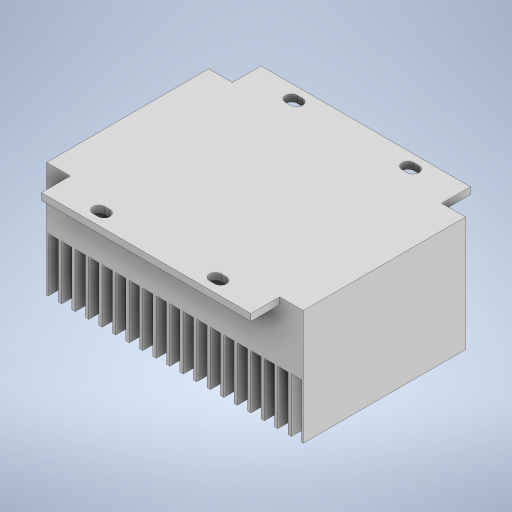
# Autodesk Inventor part: N0039 ERAM-0.01-1G-2W
Saved by Autodesk Inventor 2023 (Build 270158000, 158)
## iProperties
Created: 2023-10-03
Part Number: N0039 ERAM-0.01-1G-2W
Material: 一般
Document SubType Name: Modeling
Designer: 310611102
Density: 1 g/cm^3
Appearance: 預設
Author: 310611102
Autodesk Inventor part; units mm, degrees
ref_plane "YZ Plane" through (0, 0, 0) normal (1, 0, 0) x (0, 1, 0)
ref_plane "XZ Plane" through (0, 0, 0) normal (0, 1, 0) x (-1, 0, 0)
ref_plane "XY Plane" through (0, 0, 0) normal (0, 0, 1) x (1, 0, 0)
sketch "Sketch1" plane through (0, 0, 0) normal (0, 0, 1) x (1, 0, 0)
  line L0 (-38, 16) -> (38, 16)
  line L1 (38, 16) -> (38, -16)
  line L2 (38, -16) -> (-38, -16)
  line L3 (-38, -16) -> (-38, 16)
  line L4 (-38, 16) -> (38, -16) construction
  line L5 (38, 16) -> (-38, -16) construction
  point P0 (0, 0)
  dimension "d0" = 76
  dimension "d1" = 32
  constraints: 12 end point, 2 midpoint, 2 parallel, 1 horizontal, 1 perpendicular
  measures "d0" distance of L0.start L0.end
  measures "d1" distance of L0.end L1.end
extrude "Extrusion1" add sketch "Sketch1" along normal mid plane 48
sketch "Sketch2" plane through (-38, 16, 24) normal (0, 1, 0) x (1, 0, 0)
  line L0 (69, -8.5) -> (7, -8.5)
  line L1 (7, -8.5) -> (7, 56.5)
  line L2 (7, 56.5) -> (69, 56.5)
  line L3 (69, 56.5) -> (69, -8.5)
  line L4 (69, -8.5) -> (7, 56.5) construction
  line L5 (7, -8.5) -> (69, 56.5) construction
  line L6 (7, 48) -> (0, 48)
  line L7 (0, 48) -> (0, 0)
  line L8 (0, 0) -> (7, 0)
  line L9 (7, 0) -> (7, 48)
  line L10 (7, 48) -> (0, 0) construction
  line L11 (0, 48) -> (7, 0) construction
  line L12 (76, 48) -> (69, 48)
  line L13 (69, 48) -> (69, 0)
  line L14 (69, 0) -> (76, 0)
  line L15 (76, 0) -> (76, 48)
  line L16 (76, 48) -> (69, 0) construction
  line L17 (69, 48) -> (76, 0) construction
  line L18 (0, 48) -> (76, 48) projected
  line L19 (76, 48) -> (76, 0) projected
  line L20 (20, -4.5) -> (21.5, -4.5) construction
  line L21 (20, -6.25) -> (21.5, -6.25)
  line L22 (21.5, -2.75) -> (20, -2.75)
  arc A0 (20, -2.75) -> (20, -6.25) centre (20, -4.5) ccw
  arc A1 (21.5, -6.25) -> (21.5, -2.75) centre (21.5, -4.5) ccw
  line L23 (28.4806, 24) -> (38, 24) construction
  line L24 (38, 24) -> (38, 34.5741) construction
  line L25 (20, 52.5) -> (21.5, 52.5) construction
  line L26 (20, 54.25) -> (21.5, 54.25)
  line L27 (21.5, 50.75) -> (20, 50.75)
  arc A2 (20, 54.25) -> (20, 50.75) centre (20, 52.5) ccw
  arc A3 (21.5, 50.75) -> (21.5, 54.25) centre (21.5, 52.5) ccw
  line L28 (56, -4.5) -> (54.5, -4.5) construction
  line L29 (56, -6.25) -> (54.5, -6.25)
  line L30 (54.5, -2.75) -> (56, -2.75)
  arc A4 (56, -6.25) -> (56, -2.75) centre (56, -4.5) ccw
  arc A5 (54.5, -2.75) -> (54.5, -6.25) centre (54.5, -4.5) ccw
  line L31 (56, 54.25) -> (54.5, 54.25)
  line L32 (56, 52.5) -> (54.5, 52.5) construction
  line L33 (54.5, 50.75) -> (56, 50.75)
  arc A6 (54.5, 54.25) -> (54.5, 50.75) centre (54.5, 52.5) ccw
  arc A7 (56, 50.75) -> (56, 54.25) centre (56, 52.5) ccw
  point P0 (3.5, 24)
  point P1 (72.5, 24)
  point P2 (20.75, -4.5)
  point P3 (20.75, 52.5)
  point P4 (55.25, -4.5)
  point P5 (55.25, 52.5)
  point P6 (23.25, -4.5)
  point P7 (18.25, -4.5)
  point P8 (20.75, -6.25)
  point P9 (20.75, -2.75)
  point P10 (20.75, 52.5)
  point P11 (55.25, -4.5)
  point P12 (69, 48)
  point P13 (7, 48)
  point P14 (7, 0)
  dimension "d4" = 65
  dimension "d5" = 62
  dimension "d6" = 5
  dimension "d7" = 3.5
  dimension "d8" = 57
  dimension "d12" = 36
  constraints: 72 end point, 21 symmetric about line, 18 point on circle, 11 midpoint, 8 centre point, 7 parallel, 5 horizontal, 4 tangent, 3 collinear, 3 perpendicular, 2 point on line, 1 vertical, 6 other
  measures "d4" distance between parallel lines of L0 L2
  measures "d5" distance of L1.end L2.end
  measures "d6" distance of point (23.25, -4.5) point (18.25, -4.5)
  measures "d7" distance of point (20.75, -6.25) point (20.75, -2.75)
  measures "d8" distance of point (20.75, 52.5) point (20.75, -4.5)
  measures "d12" distance of L28.start L20.start
extrude "Extrusion2" add sketch "Sketch2" along normal blind 2
sketch "Sketch3" plane through (0, 0, 24) normal (0, 0, 1) x (1, 0, 0)
  line L0 (38, -16) -> (-38, -16) projected
  line L1 (-1.5, 0) -> (1.5, 0)
  line L2 (1.5, 0) -> (1.5, -16)
  line L3 (1.5, -16) -> (-1.5, -16)
  line L4 (-1.5, -16) -> (-1.5, 0)
  line L5 (-1.5, 0) -> (1.5, -16) construction
  line L6 (1.5, 0) -> (-1.5, -16) construction
  line L7 (-5.5, 0) -> (-2.5, 0)
  line L8 (-2.5, 0) -> (-2.5, -16)
  line L9 (-2.5, -16) -> (-5.5, -16)
  line L10 (-5.5, -16) -> (-5.5, 0)
  line L11 (-5.5, 0) -> (-2.5, -16) construction
  line L12 (-2.5, 0) -> (-5.5, -16) construction
  line L13 (-9.5, 0) -> (-6.5, 0)
  line L14 (-6.5, 0) -> (-6.5, -16)
  line L15 (-6.5, -16) -> (-9.5, -16)
  line L16 (-9.5, -16) -> (-9.5, 0)
  line L17 (-9.5, 0) -> (-6.5, -16) construction
  line L18 (-6.5, 0) -> (-9.5, -16) construction
  line L19 (-13.5, 0) -> (-10.5, 0)
  line L20 (-10.5, 0) -> (-10.5, -16)
  line L21 (-10.5, -16) -> (-13.5, -16)
  line L22 (-13.5, -16) -> (-13.5, 0)
  line L23 (-13.5, 0) -> (-10.5, -16) construction
  line L24 (-10.5, 0) -> (-13.5, -16) construction
  line L25 (-17.5, 0) -> (-14.5, 0)
  line L26 (-14.5, 0) -> (-14.5, -16)
  line L27 (-14.5, -16) -> (-17.5, -16)
  line L28 (-17.5, -16) -> (-17.5, 0)
  line L29 (-17.5, 0) -> (-14.5, -16) construction
  line L30 (-14.5, 0) -> (-17.5, -16) construction
  line L31 (2.5, 0) -> (5.5, 0)
  line L32 (5.5, 0) -> (5.5, -16)
  line L33 (5.5, -16) -> (2.5, -16)
  line L34 (2.5, -16) -> (2.5, 0)
  line L35 (2.5, 0) -> (5.5, -16) construction
  line L36 (5.5, 0) -> (2.5, -16) construction
  line L37 (-1.5, 0) -> (1.5, 0)
  line L38 (1.5, 0) -> (1.5, -16)
  line L39 (1.5, -16) -> (-1.5, -16)
  line L40 (-1.5, -16) -> (-1.5, 0)
  line L41 (-1.5, 0) -> (1.5, -16) construction
  line L42 (1.5, 0) -> (-1.5, -16) construction
  line L43 (-5.5, 0) -> (-2.5, 0)
  line L44 (-2.5, 0) -> (-2.5, -16)
  line L45 (-2.5, -16) -> (-5.5, -16)
  line L46 (-5.5, -16) -> (-5.5, 0)
  line L47 (-5.5, 0) -> (-2.5, -16) construction
  line L48 (-2.5, 0) -> (-5.5, -16) construction
  line L49 (-9.5, 0) -> (-6.5, 0)
  line L50 (-6.5, 0) -> (-6.5, -16)
  line L51 (-6.5, -16) -> (-9.5, -16)
  line L52 (-9.5, -16) -> (-9.5, 0)
  line L53 (-9.5, 0) -> (-6.5, -16) construction
  line L54 (-6.5, 0) -> (-9.5, -16) construction
  line L55 (-13.5, 0) -> (-10.5, 0)
  line L56 (-10.5, 0) -> (-10.5, -16)
  line L57 (-10.5, -16) -> (-13.5, -16)
  line L58 (-13.5, -16) -> (-13.5, 0)
  line L59 (-13.5, 0) -> (-10.5, -16) construction
  line L60 (-10.5, 0) -> (-13.5, -16) construction
  line L61 (6.5, 0) -> (9.5, 0)
  line L62 (9.5, 0) -> (9.5, -16)
  line L63 (9.5, -16) -> (6.5, -16)
  line L64 (6.5, -16) -> (6.5, 0)
  line L65 (6.5, 0) -> (9.5, -16) construction
  line L66 (9.5, 0) -> (6.5, -16) construction
  line L67 (2.5, 0) -> (5.5, 0)
  line L68 (5.5, 0) -> (5.5, -16)
  line L69 (5.5, -16) -> (2.5, -16)
  line L70 (2.5, -16) -> (2.5, 0)
  line L71 (2.5, 0) -> (5.5, -16) construction
  line L72 (5.5, 0) -> (2.5, -16) construction
  line L73 (-1.5, 0) -> (1.5, 0)
  line L74 (1.5, 0) -> (1.5, -16)
  line L75 (1.5, -16) -> (-1.5, -16)
  line L76 (-1.5, -16) -> (-1.5, 0)
  line L77 (-1.5, 0) -> (1.5, -16) construction
  line L78 (1.5, 0) -> (-1.5, -16) construction
  line L79 (-5.5, 0) -> (-2.5, 0)
  line L80 (-2.5, 0) -> (-2.5, -16)
  line L81 (-2.5, -16) -> (-5.5, -16)
  line L82 (-5.5, -16) -> (-5.5, 0)
  line L83 (-5.5, 0) -> (-2.5, -16) construction
  line L84 (-2.5, 0) -> (-5.5, -16) construction
  line L85 (-9.5, 0) -> (-6.5, 0)
  line L86 (-6.5, 0) -> (-6.5, -16)
  line L87 (-6.5, -16) -> (-9.5, -16)
  line L88 (-9.5, -16) -> (-9.5, 0)
  line L89 (-9.5, 0) -> (-6.5, -16) construction
  line L90 (-6.5, 0) -> (-9.5, -16) construction
  line L91 (10.5, 0) -> (13.5, 0)
  line L92 (13.5, 0) -> (13.5, -16)
  line L93 (13.5, -16) -> (10.5, -16)
  line L94 (10.5, -16) -> (10.5, 0)
  line L95 (10.5, 0) -> (13.5, -16) construction
  line L96 (13.5, 0) -> (10.5, -16) construction
  line L97 (6.5, 0) -> (9.5, 0)
  line L98 (9.5, 0) -> (9.5, -16)
  line L99 (9.5, -16) -> (6.5, -16)
  line L100 (6.5, -16) -> (6.5, 0)
  line L101 (6.5, 0) -> (9.5, -16) construction
  line L102 (9.5, 0) -> (6.5, -16) construction
  line L103 (2.5, 0) -> (5.5, 0)
  line L104 (5.5, 0) -> (5.5, -16)
  line L105 (5.5, -16) -> (2.5, -16)
  line L106 (2.5, -16) -> (2.5, 0)
  line L107 (2.5, 0) -> (5.5, -16) construction
  line L108 (5.5, 0) -> (2.5, -16) construction
  line L109 (-1.5, 0) -> (1.5, 0)
  line L110 (1.5, 0) -> (1.5, -16)
  line L111 (1.5, -16) -> (-1.5, -16)
  line L112 (-1.5, -16) -> (-1.5, 0)
  line L113 (-1.5, 0) -> (1.5, -16) construction
  line L114 (1.5, 0) -> (-1.5, -16) construction
  line L115 (-5.5, 0) -> (-2.5, 0)
  line L116 (-2.5, 0) -> (-2.5, -16)
  line L117 (-2.5, -16) -> (-5.5, -16)
  line L118 (-5.5, -16) -> (-5.5, 0)
  line L119 (-5.5, 0) -> (-2.5, -16) construction
  line L120 (-2.5, 0) -> (-5.5, -16) construction
  line L121 (14.5, 0) -> (17.5, 0)
  line L122 (17.5, 0) -> (17.5, -16)
  line L123 (17.5, -16) -> (14.5, -16)
  line L124 (14.5, -16) -> (14.5, 0)
  line L125 (14.5, 0) -> (17.5, -16) construction
  line L126 (17.5, 0) -> (14.5, -16) construction
  line L127 (10.5, 0) -> (13.5, 0)
  line L128 (13.5, 0) -> (13.5, -16)
  line L129 (13.5, -16) -> (10.5, -16)
  line L130 (10.5, -16) -> (10.5, 0)
  line L131 (10.5, 0) -> (13.5, -16) construction
  line L132 (13.5, 0) -> (10.5, -16) construction
  line L133 (6.5, 0) -> (9.5, 0)
  line L134 (9.5, 0) -> (9.5, -16)
  line L135 (9.5, -16) -> (6.5, -16)
  line L136 (6.5, -16) -> (6.5, 0)
  line L137 (6.5, 0) -> (9.5, -16) construction
  line L138 (9.5, 0) -> (6.5, -16) construction
  line L139 (2.5, 0) -> (5.5, 0)
  line L140 (5.5, 0) -> (5.5, -16)
  line L141 (5.5, -16) -> (2.5, -16)
  line L142 (2.5, -16) -> (2.5, 0)
  line L143 (2.5, 0) -> (5.5, -16) construction
  line L144 (5.5, 0) -> (2.5, -16) construction
  line L145 (-1.5, 0) -> (1.5, 0)
  line L146 (1.5, 0) -> (1.5, -16)
  line L147 (1.5, -16) -> (-1.5, -16)
  line L148 (-1.5, -16) -> (-1.5, 0)
  line L149 (-1.5, 0) -> (1.5, -16) construction
  line L150 (1.5, 0) -> (-1.5, -16) construction
  line L151 (-21.5, 0) -> (-18.5, 0)
  line L152 (-18.5, 0) -> (-18.5, -16)
  line L153 (-18.5, -16) -> (-21.5, -16)
  line L154 (-21.5, -16) -> (-21.5, 0)
  line L155 (-21.5, 0) -> (-18.5, -16) construction
  line L156 (-18.5, 0) -> (-21.5, -16) construction
  line L157 (-17.5, 0) -> (-14.5, 0)
  line L158 (-14.5, 0) -> (-14.5, -16)
  line L159 (-14.5, -16) -> (-17.5, -16)
  line L160 (-17.5, -16) -> (-17.5, 0)
  line L161 (-17.5, 0) -> (-14.5, -16) construction
  line L162 (-14.5, 0) -> (-17.5, -16) construction
  line L163 (-13.5, 0) -> (-10.5, 0)
  line L164 (-10.5, 0) -> (-10.5, -16)
  line L165 (-10.5, -16) -> (-13.5, -16)
  line L166 (-13.5, -16) -> (-13.5, 0)
  line L167 (-13.5, 0) -> (-10.5, -16) construction
  line L168 (-10.5, 0) -> (-13.5, -16) construction
  line L169 (-9.5, 0) -> (-6.5, 0)
  line L170 (-6.5, 0) -> (-6.5, -16)
  line L171 (-6.5, -16) -> (-9.5, -16)
  line L172 (-9.5, -16) -> (-9.5, 0)
  line L173 (-9.5, 0) -> (-6.5, -16) construction
  line L174 (-6.5, 0) -> (-9.5, -16) construction
  line L175 (-5.5, 0) -> (-2.5, 0)
  line L176 (-2.5, 0) -> (-2.5, -16)
  line L177 (-2.5, -16) -> (-5.5, -16)
  line L178 (-5.5, -16) -> (-5.5, 0)
  line L179 (-5.5, 0) -> (-2.5, -16) construction
  line L180 (-2.5, 0) -> (-5.5, -16) construction
  line L181 (-25.5, 0) -> (-22.5, 0)
  line L182 (-22.5, 0) -> (-22.5, -16)
  line L183 (-22.5, -16) -> (-25.5, -16)
  line L184 (-25.5, -16) -> (-25.5, 0)
  line L185 (-25.5, 0) -> (-22.5, -16) construction
  line L186 (-22.5, 0) -> (-25.5, -16) construction
  line L187 (-21.5, 0) -> (-18.5, 0)
  line L188 (-18.5, 0) -> (-18.5, -16)
  line L189 (-18.5, -16) -> (-21.5, -16)
  line L190 (-21.5, -16) -> (-21.5, 0)
  line L191 (-21.5, 0) -> (-18.5, -16) construction
  line L192 (-18.5, 0) -> (-21.5, -16) construction
  line L193 (-17.5, 0) -> (-14.5, 0)
  line L194 (-14.5, 0) -> (-14.5, -16)
  line L195 (-14.5, -16) -> (-17.5, -16)
  line L196 (-17.5, -16) -> (-17.5, 0)
  line L197 (-17.5, 0) -> (-14.5, -16) construction
  line L198 (-14.5, 0) -> (-17.5, -16) construction
  line L199 (-13.5, 0) -> (-10.5, 0)
  line L200 (-10.5, 0) -> (-10.5, -16)
  line L201 (-10.5, -16) -> (-13.5, -16)
  line L202 (-13.5, -16) -> (-13.5, 0)
  line L203 (-13.5, 0) -> (-10.5, -16) construction
  line L204 (-10.5, 0) -> (-13.5, -16) construction
  line L205 (-9.5, 0) -> (-6.5, 0)
  line L206 (-6.5, 0) -> (-6.5, -16)
  line L207 (-6.5, -16) -> (-9.5, -16)
  line L208 (-9.5, -16) -> (-9.5, 0)
  line L209 (-9.5, 0) -> (-6.5, -16) construction
  line L210 (-6.5, 0) -> (-9.5, -16) construction
  line L211 (-29.5, 0) -> (-26.5, 0)
  line L212 (-26.5, 0) -> (-26.5, -16)
  line L213 (-26.5, -16) -> (-29.5, -16)
  line L214 (-29.5, -16) -> (-29.5, 0)
  line L215 (-29.5, 0) -> (-26.5, -16) construction
  line L216 (-26.5, 0) -> (-29.5, -16) construction
  line L217 (-25.5, 0) -> (-22.5, 0)
  line L218 (-22.5, 0) -> (-22.5, -16)
  line L219 (-22.5, -16) -> (-25.5, -16)
  line L220 (-25.5, -16) -> (-25.5, 0)
  line L221 (-25.5, 0) -> (-22.5, -16) construction
  line L222 (-22.5, 0) -> (-25.5, -16) construction
  line L223 (-21.5, 0) -> (-18.5, 0)
  line L224 (-18.5, 0) -> (-18.5, -16)
  line L225 (-18.5, -16) -> (-21.5, -16)
  line L226 (-21.5, -16) -> (-21.5, 0)
  line L227 (-21.5, 0) -> (-18.5, -16) construction
  line L228 (-18.5, 0) -> (-21.5, -16) construction
  line L229 (-17.5, 0) -> (-14.5, 0)
  line L230 (-14.5, 0) -> (-14.5, -16)
  line L231 (-14.5, -16) -> (-17.5, -16)
  line L232 (-17.5, -16) -> (-17.5, 0)
  line L233 (-17.5, 0) -> (-14.5, -16) construction
  line L234 (-14.5, 0) -> (-17.5, -16) construction
  line L235 (-13.5, 0) -> (-10.5, 0)
  line L236 (-10.5, 0) -> (-10.5, -16)
  line L237 (-10.5, -16) -> (-13.5, -16)
  line L238 (-13.5, -16) -> (-13.5, 0)
  line L239 (-13.5, 0) -> (-10.5, -16) construction
  line L240 (-10.5, 0) -> (-13.5, -16) construction
  line L241 (-33.5, 0) -> (-30.5, 0)
  line L242 (-30.5, 0) -> (-30.5, -16)
  line L243 (-30.5, -16) -> (-33.5, -16)
  line L244 (-33.5, -16) -> (-33.5, 0)
  line L245 (-33.5, 0) -> (-30.5, -16) construction
  line L246 (-30.5, 0) -> (-33.5, -16) construction
  line L247 (-29.5, 0) -> (-26.5, 0)
  line L248 (-26.5, 0) -> (-26.5, -16)
  line L249 (-26.5, -16) -> (-29.5, -16)
  line L250 (-29.5, -16) -> (-29.5, 0)
  line L251 (-29.5, 0) -> (-26.5, -16) construction
  line L252 (-26.5, 0) -> (-29.5, -16) construction
  line L253 (-25.5, 0) -> (-22.5, 0)
  line L254 (-22.5, 0) -> (-22.5, -16)
  line L255 (-22.5, -16) -> (-25.5, -16)
  line L256 (-25.5, -16) -> (-25.5, 0)
  line L257 (-25.5, 0) -> (-22.5, -16) construction
  line L258 (-22.5, 0) -> (-25.5, -16) construction
  line L259 (-21.5, 0) -> (-18.5, 0)
  line L260 (-18.5, 0) -> (-18.5, -16)
  line L261 (-18.5, -16) -> (-21.5, -16)
  line L262 (-21.5, -16) -> (-21.5, 0)
  line L263 (-21.5, 0) -> (-18.5, -16) construction
  line L264 (-18.5, 0) -> (-21.5, -16) construction
  line L265 (-17.5, 0) -> (-14.5, 0)
  line L266 (-14.5, 0) -> (-14.5, -16)
  line L267 (-14.5, -16) -> (-17.5, -16)
  line L268 (-17.5, -16) -> (-17.5, 0)
  line L269 (-17.5, 0) -> (-14.5, -16) construction
  line L270 (-14.5, 0) -> (-17.5, -16) construction
  line L271 (-37.5, 0) -> (-34.5, 0)
  line L272 (-34.5, 0) -> (-34.5, -16)
  line L273 (-34.5, -16) -> (-37.5, -16)
  line L274 (-37.5, -16) -> (-37.5, 0)
  line L275 (-37.5, 0) -> (-34.5, -16) construction
  line L276 (-34.5, 0) -> (-37.5, -16) construction
  line L277 (-33.5, 0) -> (-30.5, 0)
  line L278 (-30.5, 0) -> (-30.5, -16)
  line L279 (-30.5, -16) -> (-33.5, -16)
  line L280 (-33.5, -16) -> (-33.5, 0)
  line L281 (-33.5, 0) -> (-30.5, -16) construction
  line L282 (-30.5, 0) -> (-33.5, -16) construction
  line L283 (-29.5, 0) -> (-26.5, 0)
  line L284 (-26.5, 0) -> (-26.5, -16)
  line L285 (-26.5, -16) -> (-29.5, -16)
  line L286 (-29.5, -16) -> (-29.5, 0)
  line L287 (-29.5, 0) -> (-26.5, -16) construction
  line L288 (-26.5, 0) -> (-29.5, -16) construction
  line L289 (-25.5, 0) -> (-22.5, 0)
  line L290 (-22.5, 0) -> (-22.5, -16)
  line L291 (-22.5, -16) -> (-25.5, -16)
  line L292 (-25.5, -16) -> (-25.5, 0)
  line L293 (-25.5, 0) -> (-22.5, -16) construction
  line L294 (-22.5, 0) -> (-25.5, -16) construction
  line L295 (-21.5, 0) -> (-18.5, 0)
  line L296 (-18.5, 0) -> (-18.5, -16)
  line L297 (-18.5, -16) -> (-21.5, -16)
  line L298 (-21.5, -16) -> (-21.5, 0)
  line L299 (-21.5, 0) -> (-18.5, -16) construction
  line L300 (-18.5, 0) -> (-21.5, -16) construction
  line L301 (18.5, 0) -> (21.5, 0)
  line L302 (21.5, 0) -> (21.5, -16)
  line L303 (21.5, -16) -> (18.5, -16)
  line L304 (18.5, -16) -> (18.5, 0)
  line L305 (18.5, 0) -> (21.5, -16) construction
  line L306 (21.5, 0) -> (18.5, -16) construction
  line L307 (14.5, 0) -> (17.5, 0)
  line L308 (17.5, 0) -> (17.5, -16)
  line L309 (17.5, -16) -> (14.5, -16)
  line L310 (14.5, -16) -> (14.5, 0)
  line L311 (14.5, 0) -> (17.5, -16) construction
  line L312 (17.5, 0) -> (14.5, -16) construction
  line L313 (10.5, 0) -> (13.5, 0)
  line L314 (13.5, 0) -> (13.5, -16)
  line L315 (13.5, -16) -> (10.5, -16)
  line L316 (10.5, -16) -> (10.5, 0)
  line L317 (10.5, 0) -> (13.5, -16) construction
  line L318 (13.5, 0) -> (10.5, -16) construction
  line L319 (6.5, 0) -> (9.5, 0)
  line L320 (9.5, 0) -> (9.5, -16)
  line L321 (9.5, -16) -> (6.5, -16)
  line L322 (6.5, -16) -> (6.5, 0)
  line L323 (6.5, 0) -> (9.5, -16) construction
  line L324 (9.5, 0) -> (6.5, -16) construction
  line L325 (2.5, 0) -> (5.5, 0)
  line L326 (5.5, 0) -> (5.5, -16)
  line L327 (5.5, -16) -> (2.5, -16)
  line L328 (2.5, -16) -> (2.5, 0)
  line L329 (2.5, 0) -> (5.5, -16) construction
  line L330 (5.5, 0) -> (2.5, -16) construction
  line L331 (-1.5, 0) -> (1.5, 0)
  line L332 (1.5, 0) -> (1.5, -16)
  line L333 (1.5, -16) -> (-1.5, -16)
  line L334 (-1.5, -16) -> (-1.5, 0)
  line L335 (-1.5, 0) -> (1.5, -16) construction
  line L336 (1.5, 0) -> (-1.5, -16) construction
  line L337 (-5.5, 0) -> (-2.5, 0)
  line L338 (-2.5, 0) -> (-2.5, -16)
  line L339 (-2.5, -16) -> (-5.5, -16)
  line L340 (-5.5, -16) -> (-5.5, 0)
  line L341 (-5.5, 0) -> (-2.5, -16) construction
  line L342 (-2.5, 0) -> (-5.5, -16) construction
  line L343 (-9.5, 0) -> (-6.5, 0)
  line L344 (-6.5, 0) -> (-6.5, -16)
  line L345 (-6.5, -16) -> (-9.5, -16)
  line L346 (-9.5, -16) -> (-9.5, 0)
  line L347 (-9.5, 0) -> (-6.5, -16) construction
  line L348 (-6.5, 0) -> (-9.5, -16) construction
  line L349 (-13.5, 0) -> (-10.5, 0)
  line L350 (-10.5, 0) -> (-10.5, -16)
  line L351 (-10.5, -16) -> (-13.5, -16)
  line L352 (-13.5, -16) -> (-13.5, 0)
  line L353 (-13.5, 0) -> (-10.5, -16) construction
  line L354 (-10.5, 0) -> (-13.5, -16) construction
  line L355 (-17.5, 0) -> (-14.5, 0)
  line L356 (-14.5, 0) -> (-14.5, -16)
  line L357 (-14.5, -16) -> (-17.5, -16)
  line L358 (-17.5, -16) -> (-17.5, 0)
  line L359 (-17.5, 0) -> (-14.5, -16) construction
  line L360 (-14.5, 0) -> (-17.5, -16) construction
  line L361 (22.5, 0) -> (25.5, 0)
  line L362 (25.5, 0) -> (25.5, -16)
  line L363 (25.5, -16) -> (22.5, -16)
  line L364 (22.5, -16) -> (22.5, 0)
  line L365 (22.5, 0) -> (25.5, -16) construction
  line L366 (25.5, 0) -> (22.5, -16) construction
  line L367 (18.5, 0) -> (21.5, 0)
  line L368 (21.5, 0) -> (21.5, -16)
  line L369 (21.5, -16) -> (18.5, -16)
  line L370 (18.5, -16) -> (18.5, 0)
  line L371 (18.5, 0) -> (21.5, -16) construction
  line L372 (21.5, 0) -> (18.5, -16) construction
  line L373 (14.5, 0) -> (17.5, 0)
  line L374 (17.5, 0) -> (17.5, -16)
  line L375 (17.5, -16) -> (14.5, -16)
  line L376 (14.5, -16) -> (14.5, 0)
  line L377 (14.5, 0) -> (17.5, -16) construction
  line L378 (17.5, 0) -> (14.5, -16) construction
  line L379 (10.5, 0) -> (13.5, 0)
  line L380 (13.5, 0) -> (13.5, -16)
  line L381 (13.5, -16) -> (10.5, -16)
  line L382 (10.5, -16) -> (10.5, 0)
  line L383 (10.5, 0) -> (13.5, -16) construction
  line L384 (13.5, 0) -> (10.5, -16) construction
  line L385 (6.5, 0) -> (9.5, 0)
  line L386 (9.5, 0) -> (9.5, -16)
  line L387 (9.5, -16) -> (6.5, -16)
  line L388 (6.5, -16) -> (6.5, 0)
  line L389 (6.5, 0) -> (9.5, -16) construction
  line L390 (9.5, 0) -> (6.5, -16) construction
  line L391 (2.5, 0) -> (5.5, 0)
  line L392 (5.5, 0) -> (5.5, -16)
  line L393 (5.5, -16) -> (2.5, -16)
  line L394 (2.5, -16) -> (2.5, 0)
  line L395 (2.5, 0) -> (5.5, -16) construction
  line L396 (5.5, 0) -> (2.5, -16) construction
  line L397 (-1.5, 0) -> (1.5, 0)
  line L398 (1.5, 0) -> (1.5, -16)
  line L399 (1.5, -16) -> (-1.5, -16)
  line L400 (-1.5, -16) -> (-1.5, 0)
  line L401 (-1.5, 0) -> (1.5, -16) construction
  line L402 (1.5, 0) -> (-1.5, -16) construction
  line L403 (-5.5, 0) -> (-2.5, 0)
  line L404 (-2.5, 0) -> (-2.5, -16)
  line L405 (-2.5, -16) -> (-5.5, -16)
  line L406 (-5.5, -16) -> (-5.5, 0)
  line L407 (-5.5, 0) -> (-2.5, -16) construction
  line L408 (-2.5, 0) -> (-5.5, -16) construction
  line L409 (-9.5, 0) -> (-6.5, 0)
  line L410 (-6.5, 0) -> (-6.5, -16)
  line L411 (-6.5, -16) -> (-9.5, -16)
  line L412 (-9.5, -16) -> (-9.5, 0)
  line L413 (-9.5, 0) -> (-6.5, -16) construction
  line L414 (-6.5, 0) -> (-9.5, -16) construction
  line L415 (-13.5, 0) -> (-10.5, 0)
  line L416 (-10.5, 0) -> (-10.5, -16)
  line L417 (-10.5, -16) -> (-13.5, -16)
  line L418 (-13.5, -16) -> (-13.5, 0)
  line L419 (-13.5, 0) -> (-10.5, -16) construction
  line L420 (-10.5, 0) -> (-13.5, -16) construction
  line L421 (26.5, 0) -> (29.5, 0)
  line L422 (29.5, 0) -> (29.5, -16)
  line L423 (29.5, -16) -> (26.5, -16)
  line L424 (26.5, -16) -> (26.5, 0)
  line L425 (26.5, 0) -> (29.5, -16) construction
  line L426 (29.5, 0) -> (26.5, -16) construction
  line L427 (22.5, 0) -> (25.5, 0)
  line L428 (25.5, 0) -> (25.5, -16)
  line L429 (25.5, -16) -> (22.5, -16)
  line L430 (22.5, -16) -> (22.5, 0)
  line L431 (22.5, 0) -> (25.5, -16) construction
  line L432 (25.5, 0) -> (22.5, -16) construction
  line L433 (18.5, 0) -> (21.5, 0)
  line L434 (21.5, 0) -> (21.5, -16)
  line L435 (21.5, -16) -> (18.5, -16)
  line L436 (18.5, -16) -> (18.5, 0)
  line L437 (18.5, 0) -> (21.5, -16) construction
  line L438 (21.5, 0) -> (18.5, -16) construction
  line L439 (14.5, 0) -> (17.5, 0)
  line L440 (17.5, 0) -> (17.5, -16)
  line L441 (17.5, -16) -> (14.5, -16)
  line L442 (14.5, -16) -> (14.5, 0)
  line L443 (14.5, 0) -> (17.5, -16) construction
  line L444 (17.5, 0) -> (14.5, -16) construction
  line L445 (10.5, 0) -> (13.5, 0)
  line L446 (13.5, 0) -> (13.5, -16)
  line L447 (13.5, -16) -> (10.5, -16)
  line L448 (10.5, -16) -> (10.5, 0)
  line L449 (10.5, 0) -> (13.5, -16) construction
  line L450 (13.5, 0) -> (10.5, -16) construction
  line L451 (6.5, 0) -> (9.5, 0)
  line L452 (9.5, 0) -> (9.5, -16)
  line L453 (9.5, -16) -> (6.5, -16)
  line L454 (6.5, -16) -> (6.5, 0)
  line L455 (6.5, 0) -> (9.5, -16) construction
  line L456 (9.5, 0) -> (6.5, -16) construction
  line L457 (2.5, 0) -> (5.5, 0)
  line L458 (5.5, 0) -> (5.5, -16)
  line L459 (5.5, -16) -> (2.5, -16)
  line L460 (2.5, -16) -> (2.5, 0)
  line L461 (2.5, 0) -> (5.5, -16) construction
  line L462 (5.5, 0) -> (2.5, -16) construction
  line L463 (-1.5, 0) -> (1.5, 0)
  line L464 (1.5, 0) -> (1.5, -16)
  line L465 (1.5, -16) -> (-1.5, -16)
  line L466 (-1.5, -16) -> (-1.5, 0)
  line L467 (-1.5, 0) -> (1.5, -16) construction
  line L468 (1.5, 0) -> (-1.5, -16) construction
  line L469 (-5.5, 0) -> (-2.5, 0)
  line L470 (-2.5, 0) -> (-2.5, -16)
  line L471 (-2.5, -16) -> (-5.5, -16)
  line L472 (-5.5, -16) -> (-5.5, 0)
  line L473 (-5.5, 0) -> (-2.5, -16) construction
  line L474 (-2.5, 0) -> (-5.5, -16) construction
  line L475 (-9.5, 0) -> (-6.5, 0)
  line L476 (-6.5, 0) -> (-6.5, -16)
  line L477 (-6.5, -16) -> (-9.5, -16)
  line L478 (-9.5, -16) -> (-9.5, 0)
  line L479 (-9.5, 0) -> (-6.5, -16) construction
  line L480 (-6.5, 0) -> (-9.5, -16) construction
  line L481 (30.5, 0) -> (33.5, 0)
  line L482 (33.5, 0) -> (33.5, -16)
  line L483 (33.5, -16) -> (30.5, -16)
  line L484 (30.5, -16) -> (30.5, 0)
  line L485 (30.5, 0) -> (33.5, -16) construction
  line L486 (33.5, 0) -> (30.5, -16) construction
  line L487 (26.5, 0) -> (29.5, 0)
  line L488 (29.5, 0) -> (29.5, -16)
  line L489 (29.5, -16) -> (26.5, -16)
  line L490 (26.5, -16) -> (26.5, 0)
  line L491 (26.5, 0) -> (29.5, -16) construction
  line L492 (29.5, 0) -> (26.5, -16) construction
  line L493 (22.5, 0) -> (25.5, 0)
  line L494 (25.5, 0) -> (25.5, -16)
  line L495 (25.5, -16) -> (22.5, -16)
  line L496 (22.5, -16) -> (22.5, 0)
  line L497 (22.5, 0) -> (25.5, -16) construction
  line L498 (25.5, 0) -> (22.5, -16) construction
  line L499 (18.5, 0) -> (21.5, 0)
  line L500 (21.5, 0) -> (21.5, -16)
  line L501 (21.5, -16) -> (18.5, -16)
  line L502 (18.5, -16) -> (18.5, 0)
  line L503 (18.5, 0) -> (21.5, -16) construction
  line L504 (21.5, 0) -> (18.5, -16) construction
  line L505 (14.5, 0) -> (17.5, 0)
  line L506 (17.5, 0) -> (17.5, -16)
  line L507 (17.5, -16) -> (14.5, -16)
  line L508 (14.5, -16) -> (14.5, 0)
  line L509 (14.5, 0) -> (17.5, -16) construction
  line L510 (17.5, 0) -> (14.5, -16) construction
  line L511 (10.5, 0) -> (13.5, 0)
  line L512 (13.5, 0) -> (13.5, -16)
  line L513 (13.5, -16) -> (10.5, -16)
  line L514 (10.5, -16) -> (10.5, 0)
  line L515 (10.5, 0) -> (13.5, -16) construction
  line L516 (13.5, 0) -> (10.5, -16) construction
  line L517 (6.5, 0) -> (9.5, 0)
  line L518 (9.5, 0) -> (9.5, -16)
  line L519 (9.5, -16) -> (6.5, -16)
  line L520 (6.5, -16) -> (6.5, 0)
  line L521 (6.5, 0) -> (9.5, -16) construction
  line L522 (9.5, 0) -> (6.5, -16) construction
  line L523 (2.5, 0) -> (5.5, 0)
  line L524 (5.5, 0) -> (5.5, -16)
  line L525 (5.5, -16) -> (2.5, -16)
  line L526 (2.5, -16) -> (2.5, 0)
  line L527 (2.5, 0) -> (5.5, -16) construction
  line L528 (5.5, 0) -> (2.5, -16) construction
  line L529 (-1.5, 0) -> (1.5, 0)
  line L530 (1.5, 0) -> (1.5, -16)
  line L531 (1.5, -16) -> (-1.5, -16)
  line L532 (-1.5, -16) -> (-1.5, 0)
  line L533 (-1.5, 0) -> (1.5, -16) construction
  line L534 (1.5, 0) -> (-1.5, -16) construction
  line L535 (-5.5, 0) -> (-2.5, 0)
  line L536 (-2.5, 0) -> (-2.5, -16)
  line L537 (-2.5, -16) -> (-5.5, -16)
  line L538 (-5.5, -16) -> (-5.5, 0)
  line L539 (-5.5, 0) -> (-2.5, -16) construction
  line L540 (-2.5, 0) -> (-5.5, -16) construction
  line L541 (34.5, 0) -> (37.5, 0)
  line L542 (37.5, 0) -> (37.5, -16)
  line L543 (37.5, -16) -> (34.5, -16)
  line L544 (34.5, -16) -> (34.5, 0)
  line L545 (34.5, 0) -> (37.5, -16) construction
  line L546 (37.5, 0) -> (34.5, -16) construction
  line L547 (30.5, 0) -> (33.5, 0)
  line L548 (33.5, 0) -> (33.5, -16)
  line L549 (33.5, -16) -> (30.5, -16)
  line L550 (30.5, -16) -> (30.5, 0)
  line L551 (30.5, 0) -> (33.5, -16) construction
  line L552 (33.5, 0) -> (30.5, -16) construction
  line L553 (26.5, 0) -> (29.5, 0)
  line L554 (29.5, 0) -> (29.5, -16)
  line L555 (29.5, -16) -> (26.5, -16)
  line L556 (26.5, -16) -> (26.5, 0)
  line L557 (26.5, 0) -> (29.5, -16) construction
  line L558 (29.5, 0) -> (26.5, -16) construction
  line L559 (22.5, 0) -> (25.5, 0)
  line L560 (25.5, 0) -> (25.5, -16)
  line L561 (25.5, -16) -> (22.5, -16)
  line L562 (22.5, -16) -> (22.5, 0)
  line L563 (22.5, 0) -> (25.5, -16) construction
  line L564 (25.5, 0) -> (22.5, -16) construction
  line L565 (18.5, 0) -> (21.5, 0)
  line L566 (21.5, 0) -> (21.5, -16)
  line L567 (21.5, -16) -> (18.5, -16)
  line L568 (18.5, -16) -> (18.5, 0)
  line L569 (18.5, 0) -> (21.5, -16) construction
  line L570 (21.5, 0) -> (18.5, -16) construction
  line L571 (14.5, 0) -> (17.5, 0)
  line L572 (17.5, 0) -> (17.5, -16)
  line L573 (17.5, -16) -> (14.5, -16)
  line L574 (14.5, -16) -> (14.5, 0)
  line L575 (14.5, 0) -> (17.5, -16) construction
  line L576 (17.5, 0) -> (14.5, -16) construction
  line L577 (10.5, 0) -> (13.5, 0)
  line L578 (13.5, 0) -> (13.5, -16)
  line L579 (13.5, -16) -> (10.5, -16)
  line L580 (10.5, -16) -> (10.5, 0)
  line L581 (10.5, 0) -> (13.5, -16) construction
  line L582 (13.5, 0) -> (10.5, -16) construction
  line L583 (6.5, 0) -> (9.5, 0)
  line L584 (9.5, 0) -> (9.5, -16)
  line L585 (9.5, -16) -> (6.5, -16)
  line L586 (6.5, -16) -> (6.5, 0)
  line L587 (6.5, 0) -> (9.5, -16) construction
  line L588 (9.5, 0) -> (6.5, -16) construction
  line L589 (2.5, 0) -> (5.5, 0)
  line L590 (5.5, 0) -> (5.5, -16)
  line L591 (5.5, -16) -> (2.5, -16)
  line L592 (2.5, -16) -> (2.5, 0)
  line L593 (2.5, 0) -> (5.5, -16) construction
  line L594 (5.5, 0) -> (2.5, -16) construction
  line L595 (-1.5, 0) -> (1.5, 0)
  line L596 (1.5, 0) -> (1.5, -16)
  line L597 (1.5, -16) -> (-1.5, -16)
  line L598 (-1.5, -16) -> (-1.5, 0)
  line L599 (-1.5, 0) -> (1.5, -16) construction
  line L600 (1.5, 0) -> (-1.5, -16) construction
  point P0 (0, 0)
  point P1 (0, -8)
  point P2 (-4, -8)
  point P3 (-8, -8)
  point P4 (-12, -8)
  point P5 (-16, -8)
  point P6 (4, -8)
  point P7 (0, -8)
  point P8 (-4, -8)
  point P9 (-8, -8)
  point P10 (-12, -8)
  point P11 (8, -8)
  point P12 (4, -8)
  point P13 (0, -8)
  point P14 (-4, -8)
  point P15 (-8, -8)
  point P16 (12, -8)
  point P17 (8, -8)
  point P18 (4, -8)
  point P19 (0, -8)
  point P20 (-4, -8)
  point P21 (16, -8)
  point P22 (12, -8)
  point P23 (8, -8)
  point P24 (4, -8)
  point P25 (0, -8)
  point P26 (-20, -8)
  point P27 (-16, -8)
  point P28 (-12, -8)
  point P29 (-8, -8)
  point P30 (-4, -8)
  point P31 (-24, -8)
  point P32 (-20, -8)
  point P33 (-16, -8)
  point P34 (-12, -8)
  point P35 (-8, -8)
  point P36 (-28, -8)
  point P37 (-24, -8)
  point P38 (-20, -8)
  point P39 (-16, -8)
  point P40 (-12, -8)
  point P41 (-32, -8)
  point P42 (-28, -8)
  point P43 (-24, -8)
  point P44 (-20, -8)
  point P45 (-16, -8)
  point P46 (-36, -8)
  point P47 (-32, -8)
  point P48 (-28, -8)
  point P49 (-24, -8)
  point P50 (-20, -8)
  point P51 (20, -8)
  point P52 (16, -8)
  point P53 (12, -8)
  point P54 (8, -8)
  point P55 (4, -8)
  point P56 (0, -8)
  point P57 (-4, -8)
  point P58 (-8, -8)
  point P59 (-12, -8)
  point P60 (-16, -8)
  point P61 (24, -8)
  point P62 (20, -8)
  point P63 (16, -8)
  point P64 (12, -8)
  point P65 (8, -8)
  point P66 (4, -8)
  point P67 (0, -8)
  point P68 (-4, -8)
  point P69 (-8, -8)
  point P70 (-12, -8)
  point P71 (28, -8)
  point P72 (24, -8)
  point P73 (20, -8)
  point P74 (16, -8)
  point P75 (12, -8)
  point P76 (8, -8)
  point P77 (4, -8)
  point P78 (0, -8)
  point P79 (-4, -8)
  point P80 (-8, -8)
  point P81 (32, -8)
  point P82 (28, -8)
  point P83 (24, -8)
  point P84 (20, -8)
  point P85 (16, -8)
  point P86 (12, -8)
  point P87 (8, -8)
  point P88 (4, -8)
  point P89 (0, -8)
  point P90 (-4, -8)
  point P91 (36, -8)
  point P92 (32, -8)
  point P93 (28, -8)
  point P94 (24, -8)
  point P95 (20, -8)
  point P96 (16, -8)
  point P97 (12, -8)
  point P98 (8, -8)
  point P99 (4, -8)
  point P100 (0, -8)
  point P101 (-1.5, -16)
  dimension "d13" = 16
  dimension "d14" = 3
  dimension "d17" = 4
  dimension "d20" = 4
  constraints: 1200 end point, 495 horizontal alignment, 398 parallel, 198 collinear, 2 midpoint, 1 horizontal, 1 perpendicular, 1 vertical alignment, 2 other
  measures "d13" distance of L1.end L2.end
  measures "d14" distance of L1.start L1.end
  measures "d17" distance of L1.start L7.start
  measures "d20" distance of L1.start L31.start
extrude "Extrusion3" cut sketch "Sketch3" against normal through all
body "Solid1"
